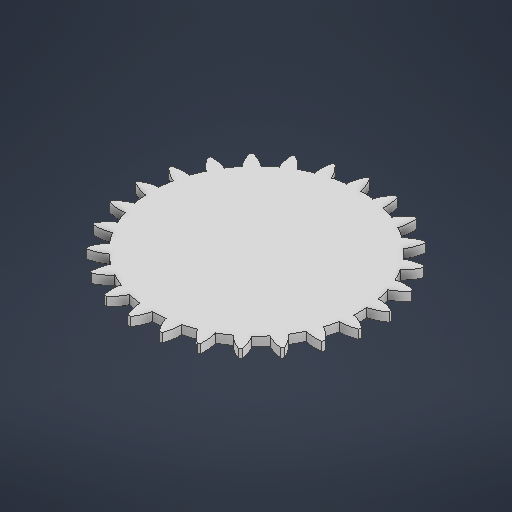
# Autodesk Inventor part: !25mm_25N_M5_Gear
Saved by Autodesk Inventor 2026.2 (Build 302298000, 298)
## iProperties
Created: 2025-12-31
Part Number: !25mm_25N_M5_Gear
Material: Generic
Document SubType Name: Modeling
Designer: Cobble
Density: 1 g/cm^3
Appearance: Default
Author: Cobble
Autodesk Inventor part; units mm, degrees
ref_plane "YZ Plane" through (0, 0, 0) normal (1, 0, 0) x (0, 1, 0)
ref_plane "XZ Plane" through (0, 0, 0) normal (0, 1, 0) x (-1, 0, 0)
ref_plane "XY Plane" through (0, 0, 0) normal (0, 0, 1) x (1, 0, 0)
sketch "Sketch2" plane through (0, 0, 0) normal (0, 0, 1) x (1, 0, 0)
  circle A0 centre (0, 0) radius 62.5 construction
  circle A1 centre (0, 0) radius 67.5
  circle A2 centre (0, 0) radius 55 construction
  circle A3 centre (0, 0) radius 58.7305
  line L0 (0, 0) -> (0, 67.5) construction
  line L1 (0, 0) -> (-16.7866, 65.3794) construction
  line L2 (0, 0) -> (-32.5184, 59.1507) construction
  line L3 (0, 0) -> (-46.2069, 49.2054) construction
  line L4 (0, 0) -> (-56.9921, 36.1683) construction
  line L5 (0, 0) -> (-64.1963, 20.8586) construction
  line L6 (0, 0) -> (-67.3668, 4.2384) construction
  line L7 (0, 0) -> (-66.3044, -12.6482) construction
  line L8 (0, 0) -> (-61.0758, -28.7401) construction
  line L9 (0, 0) -> (-52.0096, -43.0261) construction
  line L10 (0, 0) -> (-39.6755, -54.6086) construction
  line L11 (0, 0) -> (-24.8484, -62.7599) construction
  line L12 (0, 0) -> (-8.46, -66.9677) construction
  line L13 (0, 0) -> (8.46, -66.9677) construction
  line L14 (0, 0) -> (24.8484, -62.7599) construction
  line L15 (0, 0) -> (39.6755, -54.6086) construction
  line L16 (0, 0) -> (52.0096, -43.0261) construction
  line L17 (0, 0) -> (61.0758, -28.7401) construction
  line L18 (0, 0) -> (66.3044, -12.6482) construction
  line L19 (0, 0) -> (67.3668, 4.2384) construction
  line L20 (0, 0) -> (64.1963, 20.8586) construction
  line L21 (0, 0) -> (56.9921, 36.1683) construction
  line L22 (0, 0) -> (46.2069, 49.2054) construction
  line L23 (0, 0) -> (32.5184, 59.1507) construction
  line L24 (0, 0) -> (16.7866, 65.3794) construction
  line L25 (-14.6057, 56.8854) -> (-0.3094, 60.556) construction
  line L26 (-28.2936, 51.4659) -> (-2.4251, 65.6873) construction
  line L27 (-40.2038, 42.8127) -> (-7.9251, 73.1244) construction
  line L28 (-49.5878, 31.4694) -> (-17.9526, 81.3185) construction
  line L29 (-55.856, 18.1487) -> (-33.0506, 88.3367) construction
  spline S0 degree 4 poles (0, 58.7305) (0.0338, 59.877) (-2.3647, 68.8158) (-10.994, 77.9854) (-23.9392, 85.577) (-33.0506, 88.3367) knots 0 0 0 0 0 0.384291 1 1 1 1 1
  line L30 (0, 0) -> (7.3609, 58.2674) construction
  line L31 (0, 0) -> (-7.3609, 58.2674) construction
  line L32 (0, 0) -> (-21.6201, 54.6062) construction
  line L33 (0, 0) -> (-34.5209, 47.514) construction
  line L34 (0, 0) -> (-45.2526, 37.4362) construction
  line L35 (0, 0) -> (-53.1409, 25.0062) construction
  line L36 (0, 0) -> (-57.6902, 11.005) construction
  line L37 (0, 0) -> (-58.6146, -3.6877) construction
  line L38 (0, 0) -> (-55.856, -18.1487) construction
  line L39 (0, 0) -> (-49.5878, -31.4694) construction
  line L40 (0, 0) -> (-40.2038, -42.8127) construction
  line L41 (0, 0) -> (-28.2936, -51.4659) construction
  line L42 (0, 0) -> (-14.6057, -56.8854) construction
  line L43 (0, 0) -> (0, -58.7305) construction
  line L44 (0, 0) -> (14.6057, -56.8854) construction
  line L45 (0, 0) -> (28.2936, -51.4659) construction
  line L46 (0, 0) -> (40.2038, -42.8127) construction
  line L47 (0, 0) -> (49.5878, -31.4694) construction
  line L48 (0, 0) -> (55.856, -18.1487) construction
  line L49 (0, 0) -> (58.6146, -3.6877) construction
  line L50 (0, 0) -> (57.6902, 11.005) construction
  line L51 (0, 0) -> (53.1409, 25.0062) construction
  line L52 (0, 0) -> (45.2526, 37.4362) construction
  line L53 (0, 0) -> (34.5209, 47.514) construction
  line L54 (0, 0) -> (21.6201, 54.6062) construction
  line L55 (7.3609, 58.2674) -> (-7.2827, 60.1173) construction
  line L56 (21.6201, 54.6062) -> (-5.8269, 65.4733) construction
  line L57 (34.5209, 47.514) -> (-1.3024, 73.5411) construction
  line L58 (45.2526, 37.4362) -> (7.6191, 82.9273) construction
  line L59 (53.1409, 25.0062) -> (21.7184, 91.7825) construction
  spline S1 degree 4 poles (-7.3609, 58.2674) (-7.615, 59.4283) (-5.8118, 68.3898) (0.5922, 78.9773) (13.3265, 87.7784) (21.7184, 91.7825) knots 0 0 0 0 0 0.384223 1 1 1 1 1
  spline S2 degree 4 poles (-21.6201, 54.6062) (-22.155, 55.6674) (-22.6371, 64.7959) (-19.0672, 76.6434) (-8.9217, 88.3348) (-1.7893, 94.3001) knots 0 0 0 0 0 0.384223 1 1 1 1 1
  spline S3 degree 4 poles (-14.6057, 56.8854) (-14.8581, 58.0042) (-19.4042, 66.0657) (-30.0427, 72.8012) (-44.4692, 76.935) (-53.9807, 77.3421) knots 0 0 0 0 0 0.384291 1 1 1 1 1
  spline S4 degree 4 poles (-34.5209, 47.514) (-35.3029, 48.4088) (-38.04, 57.1306) (-37.5287, 69.4937) (-30.6094, 83.3409) (-25.1845, 90.8925) knots 0 0 0 0 0 0.384223 1 1 1 1 1
  spline S5 degree 4 poles (-28.2936, 51.4659) (-28.8164, 52.4869) (-35.2245, 59.1645) (-47.2038, 63.0427) (-62.2051, 63.4589) (-71.519, 61.4878) knots 0 0 0 0 0 0.384291 1 1 1 1 1
  spline S6 degree 4 poles (-45.2526, 37.4362) (-46.2326, 38.1085) (-51.0527, 45.8756) (-53.632, 57.9774) (-50.3738, 73.1103) (-46.9974, 81.7738) knots 0 0 0 0 0 0.384223 1 1 1 1 1
  spline S7 degree 4 poles (-40.2038, 42.8127) (-40.964, 43.6716) (-48.8315, 48.5458) (-61.3989, 49.323) (-76.0324, 45.9954) (-84.5635, 41.77) knots 0 0 0 0 0 0.384291 1 1 1 1 1
  spline S8 degree 4 poles (-53.1409, 25.0062) (-54.2573, 25.4137) (-60.8576, 31.738) (-66.3654, 42.8182) (-66.973, 58.286) (-65.8572, 67.517) knots 0 0 0 0 0 0.384223 1 1 1 1 1
  spline S9 degree 4 poles (-49.5878, 31.4694) (-50.5377, 32.1122) (-59.3702, 34.8767) (-71.7361, 32.5041) (-85.0823, 25.6419) (-92.2945, 19.4276) knots 0 0 0 0 0 0.384291 1 1 1 1 1
  spline S10 degree 4 poles (-57.6902, 11.005) (-58.8728, 11.122) (-66.8385, 15.6063) (-74.9289, 24.9686) (-79.3641, 39.7993) (-80.5789, 49.0178) knots 0 0 0 0 0 0.384223 1 1 1 1 1
  spline S11 degree 4 poles (-55.856, 18.1487) (-56.936, 18.5351) (-66.1784, 19.0162) (-77.5658, 13.6429) (-88.7862, 3.6772) (-94.2264, -4.1354) knots 0 0 0 0 0 0.384291 1 1 1 1 1
  spline S12 degree 4 poles (-58.6146, -3.6877) (-59.7891, -3.8685) (-68.6198, -1.5061) (-78.7843, 5.5501) (-86.7684, 18.8119) (-90.2376, 27.4386) knots 0 0 0 0 0 0.384223 1 1 1 1 1
  spline S13 degree 4 poles (-58.6146, 3.6877) (-59.7567, 3.7934) (-68.8285, 1.9609) (-78.5218, -6.0755) (-86.9113, -18.5186) (-90.2376, -27.4386) knots 0 0 0 0 0 0.384291 1 1 1 1 1
  spline S14 degree 4 poles (-55.856, -18.1487) (-56.9487, -18.6159) (-66.0894, -18.5238) (-77.6894, -14.2171) (-88.7207, -3.3576) (-94.2264, 4.1354) knots 0 0 0 0 0 0.384223 1 1 1 1 1
  spline S15 degree 4 poles (-57.6902, -11.005) (-58.8227, -11.1867) (-67.1538, -15.2176) (-74.544, -25.4122) (-79.5754, -39.5507) (-80.5789, -49.0178) knots 0 0 0 0 0 0.384291 1 1 1 1 1
  spline S16 degree 4 poles (-49.5878, -31.4694) (-50.53, -32.1936) (-59.4064, -34.3776) (-71.713, -33.0911) (-85.0984, -25.316) (-92.2945, -19.4276) knots 0 0 0 0 0 0.384223 1 1 1 1 1
  spline S17 degree 4 poles (-53.1409, -25.0062) (-54.1927, -25.4638) (-61.2595, -31.44) (-65.8823, -43.1522) (-67.2395, -58.0977) (-65.8572, -67.517) knots 0 0 0 0 0 0.384291 1 1 1 1 1
  spline S18 degree 4 poles (-40.2038, -42.8127) (-40.9362, -43.7485) (-48.9907, -48.0714) (-61.2306, -49.8857) (-76.129, -45.6838) (-84.5635, -41.77) knots 0 0 0 0 0 0.384223 1 1 1 1 1
  spline S19 degree 4 poles (-45.2526, -37.4362) (-46.1575, -38.141) (-51.5161, -45.6869) (-53.0809, -58.1807) (-50.6788, -72.9943) (-46.9974, -81.7738) knots 0 0 0 0 0 0.384291 1 1 1 1 1
  spline S20 degree 4 poles (-28.2936, -51.4659) (-28.7704, -52.5545) (-35.4967, -58.7446) (-46.9008, -63.5459) (-62.3762, -63.1811) (-71.519, -61.4878) knots 0 0 0 0 0 0.384223 1 1 1 1 1
  spline S21 degree 4 poles (-34.5209, -47.514) (-35.2221, -48.4217) (-38.5358, -57.0631) (-36.9443, -69.5536) (-30.9336, -83.3043) (-25.1845, -90.8925) knots 0 0 0 0 0 0.384291 1 1 1 1 1
  spline S22 degree 4 poles (-14.6057, -56.8854) (-14.7967, -58.0583) (-19.7723, -65.7267) (-29.6241, -73.2133) (-44.7041, -76.7084) (-53.9807, -77.3421) knots 0 0 0 0 0 0.384223 1 1 1 1 1
  spline S23 degree 4 poles (-21.6201, -54.6062) (-22.0736, -55.6598) (-23.1341, -64.8538) (-18.4864, -76.5561) (-9.2449, -88.3801) (-1.7893, -94.3001) knots 0 0 0 0 0 0.384291 1 1 1 1 1
  spline S24 degree 4 poles (0, -58.7305) (0.1067, -59.9141) (-2.8055, -68.579) (-10.486, -78.2804) (-24.223, -85.416) (-33.0506, -88.3367) knots 0 0 0 0 0 0.384223 1 1 1 1 1
  spline S25 degree 4 poles (-7.3609, -58.2674) (-7.5381, -59.4006) (-6.2788, -68.5695) (1.1331, -78.7483) (13.0248, -87.9025) (21.7184, -91.7825) knots 0 0 0 0 0 0.384291 1 1 1 1 1
  spline S26 degree 4 poles (14.6057, -56.8854) (15.0033, -58.0052) (14.3375, -67.1221) (9.3109, -78.4288) (-2.2199, -88.7565) (-10.0438, -93.7808) knots 0 0 0 0 0 0.384223 1 1 1 1 1
  spline S27 degree 4 poles (7.3609, -58.2674) (7.4711, -59.4091) (10.971, -67.9768) (20.6814, -75.9925) (34.4761, -81.9018) (43.8615, -83.4978) knots 0 0 0 0 0 0.384291 1 1 1 1 1
  spline S28 degree 4 poles (28.2936, -51.4659) (28.9573, -52.4517) (30.5797, -61.4478) (28.5229, -73.6493) (19.9227, -86.5201) (13.5941, -93.3323) knots 0 0 0 0 0 0.384223 1 1 1 1 1
  spline S29 degree 4 poles (21.6201, -54.6062) (22.0108, -55.6846) (27.5315, -63.1128) (38.9302, -68.4618) (53.7611, -70.7548) (63.2485, -69.9667) knots 0 0 0 0 0 0.384291 1 1 1 1 1
  spline S30 degree 4 poles (40.2038, -42.8127) (41.0918, -43.6025) (44.9004, -51.9124) (45.9426, -64.2421) (40.8134, -78.8473) (36.3778, -87.0194) knots 0 0 0 0 0 0.384223 1 1 1 1 1
  spline S31 degree 4 poles (34.5209, -47.514) (35.1675, -48.4613) (42.362, -54.2832) (54.7329, -56.6294) (69.6681, -55.1621) (78.6615, -52.0392) knots 0 0 0 0 0 0.384291 1 1 1 1 1
  spline S32 degree 4 poles (49.5878, -31.4694) (50.6443, -32.0135) (56.3998, -39.1152) (60.4756, -50.7984) (59.1398, -66.2203) (56.8758, -75.2387) knots 0 0 0 0 0 0.384223 1 1 1 1 1
  spline S33 degree 4 poles (45.2526, -37.4362) (46.1145, -38.193) (54.5308, -42.0428) (67.0966, -41.2387) (81.1976, -36.1033) (89.1318, -30.842) knots 0 0 0 0 0 0.384291 1 1 1 1 1
  spline S34 degree 4 poles (55.856, -18.1487) (57.0146, -18.413) (64.3555, -23.8603) (71.2087, -34.1628) (73.7501, -49.4324) (73.8, -58.7305) knots 0 0 0 0 0 0.384223 1 1 1 1 1
  spline S35 degree 4 poles (53.1409, -25.0062) (54.164, -25.5249) (63.2732, -27.1607) (75.2443, -23.2569) (87.6252, -14.7761) (94.0017, -7.7069) knots 0 0 0 0 0 0.384291 1 1 1 1 1
  spline S36 degree 4 poles (58.6146, -3.6877) (59.8025, -3.6556) (68.2675, -7.1061) (77.4675, -15.3806) (83.7264, -29.5385) (86.0871, -38.5321) knots 0 0 0 0 0 0.384223 1 1 1 1 1
  spline S37 degree 4 poles (57.6902, -11.005) (58.8101, -11.253) (68.04, -10.5719) (78.6641, -3.8138) (88.5469, 7.4797) (92.9651, 15.9125) knots 0 0 0 0 0 0.384291 1 1 1 1 1
  spline S38 degree 4 poles (57.6902, 11.005) (58.8328, 11.3315) (67.8899, 10.0946) (78.8587, 4.368) (88.4419, -7.7886) (92.9651, -15.9125) knots 0 0 0 0 0 0.384223 1 1 1 1 1
  spline S39 degree 4 poles (58.6146, 3.6877) (59.761, 3.726) (68.5315, 6.6811) (77.1412, 15.869) (83.9049, 29.2654) (86.0871, 38.5321) knots 0 0 0 0 0 0.384291 1 1 1 1 1
  spline S40 degree 4 poles (53.1409, 25.0062) (54.1665, 25.6067) (63.2466, 26.661) (75.2949, 23.8421) (87.6003, 14.4507) (94.0017, 7.7069) knots 0 0 0 0 0 0.384223 1 1 1 1 1
  spline S41 degree 4 poles (55.856, 18.1487) (56.9568, 18.4709) (64.717, 23.5142) (70.7712, 34.5547) (73.9909, 49.2123) (73.8, 58.7305) knots 0 0 0 0 0 0.384291 1 1 1 1 1
  spline S42 degree 4 poles (45.2526, 37.4362) (46.0966, 38.2728) (54.6293, 41.5522) (67.0001, 41.8181) (81.2544, 35.782) (89.1318, 30.842) knots 0 0 0 0 0 0.384223 1 1 1 1 1
  spline S43 degree 4 poles (49.5878, 31.4694) (50.5739, 32.0552) (56.836, 38.87) (59.9544, 51.0691) (59.4277, 66.067) (56.8758, 75.2387) knots 0 0 0 0 0 0.384291 1 1 1 1 1
  spline S44 degree 4 poles (34.5209, 47.514) (35.1303, 48.5342) (42.5794, 53.8325) (54.4954, 57.1666) (69.803, 54.865) (78.6615, 52.0392) knots 0 0 0 0 0 0.384223 1 1 1 1 1
  spline S45 degree 4 poles (40.2038, 42.8127) (41.0132, 43.6253) (45.3838, 51.7833) (45.3704, 64.3748) (41.1305, 78.7704) (36.3778, 87.0194) knots 0 0 0 0 0 0.384291 1 1 1 1 1
  spline S46 degree 4 poles (21.6201, 54.6062) (21.9567, 55.746) (27.8541, 62.7303) (38.5666, 68.9231) (53.9657, 70.5007) (63.2485, 69.9667) knots 0 0 0 0 0 0.384223 1 1 1 1 1
  spline S47 degree 4 poles (28.2936, 51.4659) (28.8755, 52.4544) (31.08, 61.443) (27.9357, 73.6355) (20.2489, 86.5245) (13.5941, 93.3323) knots 0 0 0 0 0 0.384291 1 1 1 1 1
  spline S48 degree 4 poles (7.3609, 58.2674) (7.4034, 59.455) (11.3786, 67.6866) (20.2145, 76.3488) (34.7374, 81.7065) (43.8615, 83.4978) knots 0 0 0 0 0 0.384223 1 1 1 1 1
  spline S49 degree 4 poles (14.6057, 56.8854) (14.9235, 57.9875) (14.8233, 67.2419) (8.7456, 78.2694) (-1.905, 88.8418) (-10.0438, 93.7808) knots 0 0 0 0 0 0.384291 1 1 1 1 1
  point P0 (-5.7407, 65.4392)
  point P1 (-22.0045, 56.4175)
  point P2 (-21.8344, 61.9556)
  point P3 (-19.5504, 70.9068)
  point P4 (-13.2434, 82.2168)
  point P5 (-15.3593, 58.5766)
  point P6 (-18.6846, 63.0205)
  point P7 (-25.8614, 68.8562)
  point P8 (-37.6117, 74.2991)
  point P9 (-35.3436, 49.1727)
  point P10 (-36.5562, 54.5792)
  point P11 (-36.57, 63.8171)
  point P12 (-33.2739, 76.3403)
  point P13 (-29.4442, 52.9166)
  point P14 (-33.7702, 56.3939)
  point P15 (-42.1728, 60.2615)
  point P16 (-54.9075, 62.6112)
  point P17 (-46.462, 38.8383)
  point P18 (-48.981, 43.7733)
  point P19 (-51.2917, 52.7176)
  point P20 (-51.2136, 65.6671)
  point P21 (-41.679, 43.9317)
  point P22 (-46.7338, 46.2239)
  point P23 (-55.8342, 47.8803)
  point P24 (-68.7532, 46.9892)
  point P25 (-54.661, 26.0635)
  point P26 (-58.3281, 30.217)
  point P27 (-62.7906, 38.3057)
  point P28 (-65.9353, 50.8677)
  point P29 (-51.2949, 32.1863)
  point P30 (-56.761, 33.1495)
  point P31 (-65.9875, 32.4907)
  point P32 (-78.279, 28.4148)
  point P33 (-59.4254, 11.651)
  point P34 (-64.0103, 14.7621)
  point P35 (-70.3442, 21.4868)
  point P36 (-76.5141, 32.8722)
  point P37 (-57.6878, 18.4186)
  point P38 (-63.2217, 17.9921)
  point P39 (-71.9945, 15.0595)
  point P40 (-82.8861, 8.0549)
  point P41 (-60.456, -3.4936)
  point P42 (-65.6705, -1.6204)
  point P43 (-73.4778, 3.3179)
  point P44 (-82.2853, 12.8111)
  point P45 (-60.456, 3.4936)
  point P46 (-65.7099, 1.7043)
  point P47 (-73.4778, -3.3179)
  point P48 (-82.2853, -12.8111)
  point P49 (-57.6878, -18.4186)
  point P50 (-63.2043, -17.9011)
  point P51 (-71.9945, -15.0595)
  point P52 (-82.8861, -8.0549)
  point P53 (-59.4254, -11.651)
  point P54 (-64.0694, -14.6907)
  point P55 (-70.3442, -21.4868)
  point P56 (-76.5141, -32.8722)
  point P57 (-51.2949, -32.1863)
  point P58 (-56.7669, -33.057)
  point P59 (-65.9875, -32.4907)
  point P60 (-78.279, -28.4148)
  point P61 (-54.661, -26.0635)
  point P62 (-58.4031, -30.1626)
  point P63 (-62.7906, -38.3057)
  point P64 (-65.9353, -50.8677)
  point P65 (-41.679, -43.9317)
  point P66 (-46.7625, -46.1358)
  point P67 (-55.8342, -47.8803)
  point P68 (-68.7532, -46.9892)
  point P69 (-46.462, -38.8383)
  point P70 (-49.0671, -43.7392)
  point P71 (-51.2917, -52.7176)
  point P72 (-51.2136, -65.6671)
  point P73 (-29.4442, -52.9166)
  point P74 (-33.8199, -56.3157)
  point P75 (-42.1728, -60.2615)
  point P76 (-54.9075, -62.6112)
  point P77 (-35.3436, -49.1727)
  point P78 (-36.6481, -54.5676)
  point P79 (-36.57, -63.8171)
  point P80 (-33.2739, -76.3403)
  point P81 (-15.3593, -58.5766)
  point P82 (-18.7522, -62.9571)
  point P83 (-25.8614, -68.8562)
  point P84 (-37.6117, -74.2991)
  point P85 (-22.0045, -56.4175)
  point P86 (-21.9263, -61.9672)
  point P87 (-19.5504, -70.9068)
  point P88 (-13.2434, -82.2168)
  point P89 (-0.3094, -60.556)
  point P90 (-2.5063, -65.6426)
  point P91 (-7.9251, -73.1244)
  point P92 (-17.9526, -81.3185)
  point P93 (-7.2827, -60.1173)
  point P94 (-5.8269, -65.4733)
  point P95 (-1.3024, -73.5411)
  point P96 (7.6191, -82.9273)
  point P97 (14.76, -58.7305)
  point P98 (13.8971, -64.2036)
  point P99 (10.5092, -72.798)
  point P100 (2.8345, -83.2284)
  point P101 (7.8966, -60.0398)
  point P102 (10.6387, -64.8654)
  point P103 (17.0275, -71.5546)
  point P104 (28.0029, -78.4272)
  point P105 (28.902, -53.2147)
  point P106 (29.4273, -58.7305)
  point P107 (28.2832, -67.8974)
  point P108 (23.4435, -79.9087)
  point P109 (22.5798, -56.1897)
  point P110 (26.4359, -60.1818)
  point P111 (34.2874, -65.072)
  point P112 (46.6272, -68.9992)
  point P113 (41.2279, -44.3552)
  point P114 (43.1085, -49.5671)
  point P115 (44.28, -58.7305)
  point P116 (42.5795, -71.568)
  point P117 (35.8442, -48.809)
  point P118 (40.5719, -51.7167)
  point P119 (49.393, -54.5007)
  point P120 (62.3218, -55.2358)
  point P121 (50.9634, -32.7088)
  point P122 (54.081, -37.2892)
  point P123 (57.4945, -45.8734)
  point P124 (59.04, -58.7305)
  point P125 (46.8564, -38.3615)
  point P126 (52.1587, -40.0021)
  point P127 (61.395, -40.5049)
  point P128 (74.1004, -38.0017)
  point P129 (57.4966, -19.0071)
  point P130 (61.6554, -22.6683)
  point P131 (67.0965, -30.1339)
  point P132 (71.7908, -42.2027)
  point P133 (54.9245, -25.5036)
  point P134 (60.4682, -25.774)
  point P135 (69.5393, -23.9641)
  point P136 (81.223, -18.3797)
  point P137 (60.4171, -4.1111)
  point P138 (65.3557, -6.6231)
  point P139 (72.4825, -12.5009)
  point P140 (80.0308, -23.0232)
  point P141 (59.5414, -11.0432)
  point P142 (64.9782, -9.9265)
  point P143 (73.3142, -5.9175)
  point P144 (83.2421, 2.397)
  point P145 (59.5414, 11.0432)
  point P146 (64.9496, 9.8383)
  point P147 (73.3142, 5.9175)
  point P148 (83.2421, -2.397)
  point P149 (60.4171, 4.1111)
  point P150 (65.4054, 6.5448)
  point P151 (72.4825, 12.5009)
  point P152 (80.0308, 23.0232)
  point P153 (54.9245, 25.5036)
  point P154 (60.4624, 25.6815)
  point P155 (69.5393, 23.9641)
  point P156 (81.223, 18.3797)
  point P157 (57.4966, 19.0071)
  point P158 (61.7229, 22.6049)
  point P159 (67.0965, 30.1339)
  point P160 (71.7908, 42.2027)
  point P161 (46.8564, 38.3615)
  point P162 (52.1761, 39.9111)
  point P163 (61.395, 40.5049)
  point P164 (74.1004, 38.0017)
  point P165 (50.9634, 32.7088)
  point P166 (54.1622, 37.2446)
  point P167 (57.4945, 45.8734)
  point P168 (59.04, 58.7305)
  point P169 (35.8442, 48.809)
  point P170 (40.6114, 51.6329)
  point P171 (49.393, 54.5007)
  point P172 (62.3218, 55.2358)
  point P173 (41.2279, 44.3552)
  point P174 (43.1983, 49.544)
  point P175 (44.28, 58.7305)
  point P176 (42.5795, 71.568)
  point P177 (22.5798, 56.1897)
  point P178 (26.495, 60.1104)
  point P179 (34.2874, 65.072)
  point P180 (46.6272, 68.9992)
  point P181 (28.902, 53.2147)
  point P182 (29.52, 58.7305)
  point P183 (28.2832, 67.8974)
  point P184 (23.4435, 79.9087)
  point P185 (7.8966, 60.0398)
  point P186 (10.7137, 64.8109)
  point P187 (17.0275, 71.5546)
  point P188 (28.0029, 78.4272)
  point P189 (14.76, 58.7305)
  point P190 (13.9869, 64.2267)
  point P191 (10.5092, 72.798)
  point P192 (2.8345, 83.2284)
  point P193 (58.6146, 3.6877)
  point P194 (67.0639, 7.6601)
  point P195 (66.8764, 9.1544)
  point P196 (57.6902, 11.005)
  point P197 (55.856, 18.1487)
  point P198 (63.052, 24.0976)
  point P199 (62.4987, 25.4983)
  dimension "d10" = 135
  dimension "d12" = 117.461
  dimension "d9" = 125
  dimension "d11" = 110
  dimension "d15" = 360
  dimension "d17" = 14.76
  dimension "d18" = 29.52
  dimension "d19" = 44.28
  dimension "d20" = 59.04
  dimension "d21" = 73.8
  dimension "d24" = 360
  dimension "d26" = 14.76
  dimension "d27" = 29.52
  dimension "d28" = 44.28
  dimension "d29" = 59.04
  dimension "d30" = 73.8
  dimension "d33" = 360
  constraints: 120 end point, 8 point on line, 5 perpendicular, 4 coincident, 2 centre point, 1 vertical, 825 other
  measures "d9" diameter of A0
  measures "d11" diameter of A2
  measures "d17" distance of L25.start L25.end
  measures "d18" distance of L26.start L26.end
  measures "d19" distance of L27.start L27.end
  measures "d20" distance of L28.start L28.end
  measures "d21" distance of L29.start L29.end
  measures "d26" distance of L30.end L55.end
  measures "d27" distance of L54.end L56.end
  measures "d28" distance of L53.end L57.end
  measures "d29" distance of L52.end L58.end
  measures "d30" distance of L51.end L59.end
extrude "Extrusion1" add sketch "Sketch2" along normal blind 5 contours S39 A3 S38 A1 | A1 S37 A3 S36 | A3 | S41 A3 S40 A1 | A1 S35 A3 S34 | S43 A3 S42 A1 | A1 S33 A3 S32 | S45 A3 S44 A1 | A1 S31 A3 S30 | S47 A3 S46 A1 | A1 S29 A3 S28 | S49 A3 S48 A1 | A1 S27 A3 S26 | S0 A3 S1 A1 | A1 S25 A3 S24 | S3 A3 S2 A1 | A1 S23 A3 S22 | S5 A3 S4 A1 | A1 S21 A3 S20 | S7 A3 S6 A1 | A1 S19 A3 S18 | S9 A3 S8 A1 | A1 S17 A3 S16 | S11 A3 S10 A1 | A1 S15 A3 S14 | S13 A3 S12 A1
equation "\"d18\" = 2 * d17"
equation "\"d19\" = 3 * d17"
equation "\"d20\" = 4 * d17"
equation "\"d21\" = 5 * d17"
equation "\"d26\" = d17"
equation "\"d27\" = 2 * d17"
equation "\"d28\" = 3 * d17"
equation "\"d29\" = 4 * d17"
equation "\"d30\" = 5 * d17"
body "Solid1"
